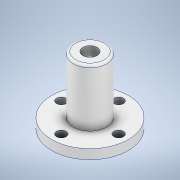
# Autodesk Inventor part: pintle body
Saved by Autodesk Inventor 2021 (Build 250183000, 183)
## iProperties
Created: 2022-07-06
Part Number: pintle body
Material: Aluminum 6061
Document SubType Name: Modeling
Designer: pc
Density: 2.7 g/cm^3
Appearance: Aluminum - Flat
Mass: 248.903 g
Surface Area: 225.862 cm^2
Volume: 92.1863 cm^3
Author: pc
Autodesk Inventor part; units mm, degrees
ref_plane "YZ Plane" through (0, 0, 0) normal (1, 0, 0) x (0, 1, 0)
ref_plane "XY Plane" through (0, 0, 0) normal (0, 0, 1) x (1, 0, 0)
sketch "Sketch1" plane through (0, 0, 0) normal (0, 1, 0) x (-1, 0, 0)
  circle A0 centre (0, 0) radius 40
  circle A1 centre (0, -30) radius 5
  circle A2 centre (30, 0) radius 5
  circle A3 centre (0, 30) radius 5
  circle A4 centre (-30, 0) radius 5
  dimension "d0" = 80
  dimension "d1" = 10
  dimension "d2" = 30
  dimension "d5" = 360
  constraints: 5 centre point, 1 coincident, 9 other
  measures "d0" diameter of A0
  measures "d1" diameter of A1
  measures "d2" distance of A1.centre point (0, 0)
extrude "Extrusion1" add sketch "Sketch1" along normal blind 10
thread "Thread1" size "M10x1.5" class "6H" standard "ANSI Metric M Profile" length 20
thread "Thread2" size "M10x1.5" class "6H" standard "ANSI Metric M Profile" length 20
thread "Thread3" size "M10x1.5" class "6H" standard "ANSI Metric M Profile" length 20
thread "Thread4" size "M10x1.5" class "6H" standard "ANSI Metric M Profile" length 20
sketch "Sketch2" plane through (0, 10, 0) normal (0, 1, 0) x (1, 0, 0)
  circle A0 centre (0, 0) radius 17.5
  dimension "d17" = 35
  constraints: 1 centre point, 1 coincident
  measures "d17" diameter of A0
extrude "Extrusion2" add sketch "Sketch2" along normal blind 59.807
sketch "Sketch3" plane through (0, 69.807, 0) normal (0, 1, 0) x (1, 0, 0)
  circle A0 centre (0, 0) radius 10
  dimension "d20" = 20
  constraints: 1 centre point, 1 coincident
  measures "d20" diameter of A0
hole "Hole1" at (0, 69.807, 0) direction (0, -1, 0) diameter 15 end through all
ref_plane "Work Plane1" through (0, 68, 0) normal (0, 1, 0) x (-1, 0, 0)
ref_plane "Work Plane2" through (0, 65, 0) normal (0, -1, 0) x (1, 0, 0)
sketch "Sketch6" plane through (0, 65, 0) normal (0, -1, 0) x (1, 0, 0)
  point P0 (0, 0)
fillet "Fillet2" radius 2.5 1 edges at (-17.5, 69.807, 0)
thread "Thread10" size "M15x1.5" class "6H" standard "ANSI Metric M Profile" length 16.401
body "Solid1"
